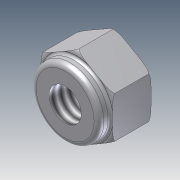
# Autodesk Inventor part: HW-00002
Saved by Autodesk Inventor 2012 (Build 160160000, 160)
## iProperties
Created: 2008-05-01
Part Number: HW-00002
Document SubType Name: Modeling
Designer: dfoster
Density: 1 g/cm^3
Description: Nut, Lock 1/4-20
Mass: 0.637638 g
Surface Area: 5.6464 cm^2
Volume: 0.637638 cm^3
Material: Default
Title: Nut, Lock 1/4-20
Author: dfoster
Autodesk Inventor part; units mm, degrees
ref_plane "YZ Plane" through (0, 0, 0) normal (1, 0, 0) x (0, 1, 0)
ref_plane "XZ Plane" through (0, 0, 0) normal (0, 1, 0) x (-1, 0, 0)
sketch "Sketch1" plane through (0, 0, 0) normal (0, 0, 1) x (1, 0, 0)
  line L0 (-12.7, 6.2842) -> (-18.2562, 9.4921)
  line L1 (-18.2562, 9.4921) -> (-18.2563, 15.9079)
  line L2 (-18.2563, 15.9079) -> (-12.7, 19.1158)
  line L3 (-12.7, 19.1158) -> (-7.1438, 15.9079)
  line L4 (-7.1438, 15.9079) -> (-7.1438, 9.4921)
  line L5 (-7.1438, 9.4921) -> (-12.7, 6.2842)
  point P0 (-12.7, 12.7)
  dimension "d0" = 11.1125
  constraints: 12 end point, 13 other
  measures "d0" distance between parallel lines of L5 L2
extrude "Extrusion1" add sketch "Sketch1" along normal blind 5.969
ref_plane "Work Plane1" through (-12.7, 19.1158, 5.969) normal (-1, 0, 0) x (0, 0, -1)
sketch "Sketch3" plane through (-12.7, 19.1158, 5.969) normal (-1, 0, 0) x (0, 0, -1)
  line L0 (0, 12.8316) -> (5.969, 12.8316) projected
  line L1 (5.969, 12.8316) -> (5.969, 0) projected
  line L2 (5.969, 0) -> (0, 0) projected
  line L3 (0, 0) -> (0, 12.8316) projected
  line L4 (0, 12.0696) -> (0, 6.4158)
  line L5 (0, 6.4158) -> (5.969, 6.4158)
  line L6 (5.969, 6.4158) -> (5.969, 12.0696)
  arc A0 (5.969, 12.0696) -> (5.625, 12.8316) centre (4.953, 12.0696) ccw
  arc A1 (0.344, 12.8316) -> (0, 12.0696) centre (1.016, 12.0696) ccw
  line L7 (0.344, 12.8316) -> (5.625, 12.8316)
  line L8 (5.969, 12.8316) -> (5.969, 9.6237) projected
  line L9 (0, 12.8316) -> (0, 9.6237) projected
  line L10 (0, 9.6237) -> (0, 3.2079) projected
  dimension "d4" = 1.016
  dimension "d5" = 0.762
  dimension "d6" = 0.762
  constraints: 8 end point, 4 point on circle, 3 collinear, 2 centre point, 2 horizontal, 2 tangent, 1 equal radius, 1 midpoint, 1 perpendicular, 1 point on line, 1 vertical
  measures "d4" radius of A1
  measures "d5" distance from line of A1.centre L7
  measures "d6" distance from line of L7 A0.centre
revolve "Revolution1" cut sketch "Sketch3" angle 360 about axis through (-12.7, 12.7, 5.969) along (0, 0, -1) keep common part contours L0 A0 L1 L5 L3 A1
sketch "Sketch4" plane through (0, 0, 5.969) normal (0, 0, 1) x (1, 0, 0)
  arc A0 (-16.3838, 16.989) -> (-18.2562, 13.7458) centre (-12.7, 12.7) ccw projected
  circle A1 centre (-12.7, 12.7) radius 5.2451
  dimension "d8" = 10.4902
  constraints: 1 centre point, 1 concentric
  measures "d8" diameter of A1
extrude "Extrusion2" add sketch "Sketch4" along normal blind 1.778
fillet "Fillet1" radius 0.762 1 edges at (-17.9451, 12.7, 7.747)
fillet "Fillet2" radius 0.381 1 edges at (-17.9451, 12.7, 5.969)
hole "Hole1" at (-12.7, 12.7, 7.747) direction (0, 0, -1) diameter 4.9784 end through all thread size "1/4-20 UNC" class "2B" standard "ANSI Unified Screw Threads"
body "Solid1"
